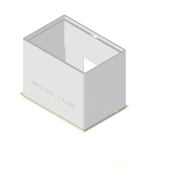
# Autodesk Inventor part: NematostellaImager_v0
Saved by Autodesk Inventor 2022.5 (Build 265521000, 521)
## iProperties
Created: 2023-11-03
Part Number: NematostellaImager_v0
Material: Generisch
Document SubType Name: Modeling
Designer: diederichbenedict
Density: 1 g/cm^3
Appearance: Vorgabe
Author: diederichbenedict
Autodesk Inventor part; units mm, degrees
ref_plane "Arbeitsebene1" through (-165.0574, -46.7107, -74.5227) normal (0, -1, 0) x (1, 0, 0)
sketch "Skizze1" plane through (-165.0574, -46.7107, -74.5227) normal (0, -1, 0) x (1, 0, 0)
  arc A0 (-60.945, 42.8) -> (-63.945, 39.8) centre (-60.945, 39.8) ccw projected
  arc A1 (60.945, -42.8) -> (63.945, -39.8) centre (60.945, -39.8) ccw projected
  line L0 (-61.445, 40.3) -> (61.445, 40.3)
  line L1 (61.445, 40.3) -> (61.445, -40.3)
  line L2 (61.445, -40.3) -> (-61.445, -40.3)
  line L3 (-61.445, -40.3) -> (-61.445, 40.3)
  line L4 (66.445, 45.3) -> (-66.445, 45.3)
  line L5 (-66.445, 45.3) -> (-66.445, -45.3)
  line L6 (-66.445, -45.3) -> (66.445, -45.3)
  line L7 (66.445, -45.3) -> (66.445, 45.3)
  circle A2 centre (14.5, -91.1) radius 3 projected
  circle A3 centre (-20.8, -84.8) radius 3 projected
  circle A4 centre (-14.5, -49.5) radius 3 projected
  circle A5 centre (20.8, -55.8) radius 3 projected
  circle A6 centre (14.5, -49.5) radius 3 projected
  circle A7 centre (-20.8, -55.8) radius 3 projected
  circle A8 centre (-14.5, -91.1) radius 3 projected
  circle A9 centre (20.8, -84.8) radius 3 projected
  line L8 (15, -87.3) -> (-15, -87.3) projected
  arc A10 (15, -87.3) -> (17, -85.3) centre (15, -85.3) ccw projected
  line L9 (17, -85.3) -> (17, -55.3) projected
  arc A11 (17, -55.3) -> (15, -53.3) centre (15, -55.3) ccw projected
  line L10 (-15, -53.3) -> (15, -53.3) projected
  arc A12 (-15, -53.3) -> (-17, -55.3) centre (-15, -55.3) ccw projected
  line L11 (-17, -55.3) -> (-17, -85.3) projected
  arc A13 (-17, -85.3) -> (-15, -87.3) centre (-15, -85.3) ccw projected
  circle A14 centre (21, -91.3) radius 2.5 projected
  circle A15 centre (-21, -49.3) radius 2.5 projected
  circle A16 centre (21, -49.3) radius 2.5 projected
  circle A17 centre (-21, -91.3) radius 2.5 projected
  line L12 (-24.25, -47.3) -> (-24.25, -66.05) projected
  arc A18 (-23, -46.05) -> (-24.25, -47.3) centre (-23, -47.3) ccw projected
  line L13 (-4.25, -46.05) -> (-23, -46.05) projected
  line L14 (-4.25, -43.9226) -> (-4.25, -46.05) projected
  arc A19 (-4.25, -43.9226) -> (-5.0944, -42.9348) centre (-5.25, -43.9226) ccw projected
  arc A20 (-4.9, -40.45) -> (-5.0944, -42.9348) centre (-4.9, -41.7) ccw projected
  line L15 (4.9, -40.45) -> (-4.9, -40.45) projected
  arc A21 (5.0944, -42.9348) -> (4.9, -40.45) centre (4.9, -41.7) ccw projected
  arc A22 (5.0944, -42.9348) -> (4.25, -43.9226) centre (5.25, -43.9226) ccw projected
  line L16 (4.25, -46.05) -> (4.25, -43.9226) projected
  line L17 (23, -46.05) -> (4.25, -46.05) projected
  arc A23 (24.25, -47.3) -> (23, -46.05) centre (23, -47.3) ccw projected
  line L18 (24.25, -64.2875) -> (24.25, -47.3) projected
  arc A24 (24.056, -64.3217) -> (24.25, -64.2875) centre (24.15, -64.2875) ccw projected
  arc A25 (24.056, -64.3217) -> (18.8, -65.25) centre (21.51, -65.25) ccw projected
  line L19 (18.8, -75.35) -> (18.8, -65.25) projected
  arc A26 (18.8, -75.35) -> (24.056, -76.2783) centre (21.51, -75.35) ccw projected
  arc A27 (24.25, -76.3125) -> (24.056, -76.2783) centre (24.15, -76.3125) ccw projected
  line L20 (24.25, -93.3) -> (24.25, -76.3125) projected
  arc A28 (23, -94.55) -> (24.25, -93.3) centre (23, -93.3) ccw projected
  line L21 (6.0125, -94.55) -> (23, -94.55) projected
  arc A29 (5.9783, -94.356) -> (6.0125, -94.55) centre (6.0125, -94.45) ccw projected
  arc A30 (5.9783, -94.356) -> (5.05, -89.1) centre (5.05, -91.81) ccw projected
  line L22 (-5.05, -89.1) -> (5.05, -89.1) projected
  arc A31 (-5.05, -89.1) -> (-5.9783, -94.356) centre (-5.05, -91.81) ccw projected
  arc A32 (-6.0125, -94.55) -> (-5.9783, -94.356) centre (-6.0125, -94.45) ccw projected
  line L23 (-23, -94.55) -> (-6.0125, -94.55) projected
  arc A33 (-24.25, -93.3) -> (-23, -94.55) centre (-23, -93.3) ccw projected
  line L24 (-24.25, -74.55) -> (-24.25, -93.3) projected
  line L25 (-26.3774, -74.55) -> (-24.25, -74.55) projected
  arc A34 (-26.3774, -74.55) -> (-27.3652, -75.3944) centre (-26.3774, -75.55) ccw projected
  arc A35 (-29.85, -75.2) -> (-27.3652, -75.3944) centre (-28.6, -75.2) ccw projected
  line L26 (-29.85, -65.4) -> (-29.85, -75.2) projected
  arc A36 (-27.3652, -65.2056) -> (-29.85, -65.4) centre (-28.6, -65.4) ccw projected
  arc A37 (-27.3652, -65.2056) -> (-26.3774, -66.05) centre (-26.3774, -65.05) ccw projected
  line L27 (-24.25, -66.05) -> (-26.3774, -66.05) projected
  line L28 (-25, -65.3) -> (-25, -47.3) projected
  line L29 (-25, -65.3) -> (-25, -47.3)
  arc A38 (-23, -45.3) -> (-25, -47.3) centre (-23, -47.3) ccw
  line L30 (-23, -45.3) -> (-5, -45.3)
  line L31 (-5, -45.3) -> (-5, -43.9226)
  arc A39 (-5, -43.9226) -> (-5.2111, -43.6757) centre (-5.25, -43.9226) ccw
  arc A40 (-4.9, -39.7) -> (-5.2111, -43.6757) centre (-4.9, -41.7) ccw
  line L32 (-4.9, -39.7) -> (4.9, -39.7)
  arc A41 (5.2111, -43.6757) -> (4.9, -39.7) centre (4.9, -41.7) ccw
  arc A42 (5.2111, -43.6757) -> (5, -43.9226) centre (5.25, -43.9226) ccw
  line L33 (5, -43.9226) -> (5, -45.3)
  line L34 (5, -45.3) -> (23, -45.3)
  arc A43 (25, -47.3) -> (23, -45.3) centre (23, -47.3) ccw
  line L35 (25, -47.3) -> (25, -64.2875)
  arc A44 (23.3514, -64.5786) -> (25, -64.2875) centre (24.15, -64.2875) ccw
  arc A45 (23.3514, -64.5786) -> (19.55, -65.25) centre (21.51, -65.25) ccw
  line L36 (19.55, -65.25) -> (19.55, -75.35)
  arc A46 (19.55, -75.35) -> (23.3514, -76.0214) centre (21.51, -75.35) ccw
  arc A47 (25, -76.3125) -> (23.3514, -76.0214) centre (24.15, -76.3125) ccw
  line L37 (25, -76.3125) -> (25, -93.3)
  arc A48 (23, -95.3) -> (25, -93.3) centre (23, -93.3) ccw
  line L38 (23, -95.3) -> (6.0125, -95.3)
  arc A49 (5.7214, -93.6514) -> (6.0125, -95.3) centre (6.0125, -94.45) ccw
  arc A50 (5.7214, -93.6514) -> (5.05, -89.85) centre (5.05, -91.81) ccw
  line L39 (5.05, -89.85) -> (-5.05, -89.85)
  arc A51 (-5.05, -89.85) -> (-5.7214, -93.6514) centre (-5.05, -91.81) ccw
  arc A52 (-6.0125, -95.3) -> (-5.7214, -93.6514) centre (-6.0125, -94.45) ccw
  line L40 (-6.0125, -95.3) -> (-23, -95.3)
  arc A53 (-25, -93.3) -> (-23, -95.3) centre (-23, -93.3) ccw
  line L41 (-25, -93.3) -> (-25, -75.3)
  line L42 (-25, -75.3) -> (-26.3774, -75.3)
  arc A54 (-26.3774, -75.3) -> (-26.6243, -75.5111) centre (-26.3774, -75.55) ccw
  arc A55 (-30.6, -75.2) -> (-26.6243, -75.5111) centre (-28.6, -75.2) ccw
  line L43 (-30.6, -75.2) -> (-30.6, -65.4)
  arc A56 (-26.6243, -65.0889) -> (-30.6, -65.4) centre (-28.6, -65.4) ccw
  arc A57 (-26.6243, -65.0889) -> (-26.3774, -65.3) centre (-26.3774, -65.05) ccw
  line L44 (-26.3774, -65.3) -> (-25, -65.3)
  point P0 (165.0574, 74.5227)
  point P1 (0, -45.3)
  point P2 (5, -45.3)
  point P3 (-5, -45.3)
  dimension "d0" = 5
  dimension "d16" = 0.5
  dimension "d20" = 0.5
  dimension "d21" = 0.5
  dimension "d22" = 0.5
  constraints: 48 end point, 40 point on circle, 20 centre point, 4 parallel, 2 perpendicular, 1 horizontal, 1 midpoint, 38 other
  measures "d0" distance between parallel lines of L0 L4
  measures "d16" vertical distance of A0.end L0.start
  measures "d20" horizontal distance of L0.start A0.start
  measures "d21" horizontal distance of A1.start L1.end
  measures "d22" vertical distance of A1.end L1.end
extrude "Extrusion1" add sketch "Skizze1" along normal blind 5 contours L3 L2 A40 A39 L31 L6 L5 L4 L7 L33 A42 A41 L1 L0 | L0 L1 L2 A41 L32 A40 L3
sketch "Skizze2" plane through (-165.0574, -46.7107, -74.5227) normal (0, -1, 0) x (1, 0, 0)
  point P0 (165.0574, 74.5227)
sketch "Skizze4" plane through (-165.0574, -46.7107, -74.5227) normal (0, 1, 0) x (1, 0, 0)
  line L0 (-66.445, 45.3) -> (-5, 45.3) projected
  line L1 (-66.445, -45.3) -> (-66.445, 45.3) projected
  line L2 (66.445, -45.3) -> (-66.445, -45.3) projected
  line L3 (66.445, 45.3) -> (66.445, -45.3) projected
  line L4 (-62.445, 43.3) -> (-20, 43.3)
  line L5 (21, 42.3) -> (62.445, 42.3)
  line L6 (62.445, 42.3) -> (62.445, -41.3)
  line L7 (62.445, -41.3) -> (-62.445, -41.3)
  line L8 (-62.445, -41.3) -> (-62.445, 43.3)
  line L9 (-25, 46.3) -> (-25, 43.3)
  line L10 (-4.9, 39.7) -> (4.9, 39.7) projected
  arc A0 (-5.2111, 43.6757) -> (-4.9, 39.7) centre (-4.9, 41.7) ccw projected
  arc A1 (-5.2111, 43.6757) -> (-5, 43.9226) centre (-5.25, 43.9226) ccw projected
  line L11 (-5, 45.3) -> (-5, 43.9226) projected
  line L12 (5, 45.3) -> (66.445, 45.3) projected
  line L13 (5, 43.9226) -> (5, 45.3) projected
  arc A2 (5, 43.9226) -> (5.2111, 43.6757) centre (5.25, 43.9226) ccw projected
  arc A3 (4.9, 39.7) -> (5.2111, 43.6757) centre (4.9, 41.7) ccw projected
  line L14 (-25, 66.3) -> (-25, 48.3)
  line L15 (25, 48.3) -> (25, 65.2875)
  line L16 (25, 48.3) -> (25, 42.3)
  line L17 (-25, 43.3) -> (-25, 46.3)
  point P0 (165.0574, -74.5227)
  point P1 (-25, 45.3)
  point P2 (25, 45.3)
  dimension "d9" = 4
  constraints: 20 end point, 2 perpendicular, 2 point on line, 2 vertical, 1 parallel, 6 other
  measures "d9" distance between parallel lines of L1 L8
ref_plane "Arbeitsebene2" through (-229.0024, 13.2893, -117.3227) normal (0, -1, 0) x (1, 0, 0)
ref_plane "Arbeitsebene3" through (-231.5024, 51.2893, -119.8227) normal (0, 1, 0) x (0, 0, 1)
extrude "Extrusion2" add sketch "Skizze4" along normal up to surface (98 mm away) contours L0 L9 L4 L8 L7 L6 L5 L16 L12 L3 L2 L1
sketch "Skizze5" plane through (-231.5024, 51.2893, -29.2227) normal (0, 1, 0) x (1, 0, 0)
  line L0 (5.5, 2.5) -> (127.39, 2.5) projected
  arc A0 (127.39, 2.5) -> (130.39, 5.5) centre (127.39, 5.5) ccw projected
  line L1 (130.39, 5.5) -> (130.39, 85.1) projected
  arc A1 (130.39, 85.1) -> (127.39, 88.1) centre (127.39, 85.1) ccw projected
  line L2 (127.39, 88.1) -> (5.5, 88.1) projected
  arc A2 (5.5, 88.1) -> (2.5, 85.1) centre (5.5, 85.1) ccw projected
  line L3 (2.5, 85.1) -> (2.5, 5.5) projected
  arc A3 (2.5, 5.5) -> (5.5, 2.5) centre (5.5, 5.5) ccw projected
  line L4 (15.2426, 4) -> (125.89, 4) projected
  arc A4 (13.1213, 4.8787) -> (15.2426, 4) centre (15.2426, 7) ccw projected
  line L5 (13.1213, 4.8787) -> (4.8787, 13.1213) projected
  arc A5 (4, 15.2426) -> (4.8787, 13.1213) centre (7, 15.2426) ccw projected
  line L6 (4, 75.3574) -> (4, 15.2426) projected
  arc A6 (4.8787, 77.4787) -> (4, 75.3574) centre (7, 75.3574) ccw projected
  line L7 (4.8787, 77.4787) -> (13.1213, 85.7213) projected
  arc A7 (15.2426, 86.6) -> (13.1213, 85.7213) centre (15.2426, 83.6) ccw projected
  line L8 (125.89, 86.6) -> (15.2426, 86.6) projected
  arc A8 (128.89, 83.6) -> (125.89, 86.6) centre (125.89, 83.6) ccw projected
  line L9 (128.89, 7) -> (128.89, 83.6) projected
  arc A9 (125.89, 4) -> (128.89, 7) centre (125.89, 7) ccw projected
  line L10 (0, 0) -> (0, 90.6) construction
  line L11 (132.89, 0) -> (0, 0) construction
  line L12 (132.89, 90.6) -> (132.89, 0) construction
  line L13 (91.445, 90.6) -> (132.89, 90.6) construction
  line L14 (91.445, 87.6) -> (91.445, 90.6) construction
  line L15 (128.89, 87.6) -> (91.445, 87.6) construction
  line L16 (128.89, 4) -> (128.89, 87.6) construction
  line L17 (4, 4) -> (128.89, 4) construction
  line L18 (4, 88.6) -> (4, 4) construction
  line L19 (41.445, 88.6) -> (4, 88.6) construction
  line L20 (41.445, 90.6) -> (41.445, 88.6) construction
  line L21 (0, 90.6) -> (41.445, 90.6) construction
  line L22 (0, 90.6) -> (132.89, 90.6)
  line L23 (132.89, 90.6) -> (132.89, 0)
  line L24 (132.89, 0) -> (0, 0)
  line L25 (0, 0) -> (0, 90.6)
  point P0 (231.5024, -29.2227)
  constraints: 8 end point, 2 parallel, 1 horizontal, 1 perpendicular
extrude "Extrusion3" add sketch "Skizze5" along normal blind 5 contours L22 L23 L24 L25
sketch "Skizze6" plane through (-227.5024, 51.2893, -33.2732) normal (0, 1, 0) x (1, 0, 0)
  point P0 (227.5024, -33.2732)
ref_plane "Arbeitsebene4" through (-189.5574, 3.2893, -169.3472) normal (0, 1, 0) x (0, 0, 1)
sketch "Skizze7" plane through (-227.5024, 51.2893, -34.0644) normal (0, 1, 0) x (1, 0, 0)
  arc A0 (-1.5, 0.6583) -> (1.5, -2.3417) centre (1.5, 0.6583) ccw projected
  line L0 (1.5, -2.3417) -> (123.39, -2.3417) projected
  arc A1 (123.39, -2.3417) -> (126.39, 0.6583) centre (123.39, 0.6583) ccw projected
  line L1 (126.39, 0.6583) -> (126.39, 80.2583) projected
  arc A2 (126.39, 80.2583) -> (123.39, 83.2583) centre (123.39, 80.2583) ccw projected
  line L2 (123.39, 83.2583) -> (87.445, 83.2583) projected
  line L3 (87.445, 82.7583) -> (87.445, 83.2583) projected
  line L4 (124.89, 82.7583) -> (87.445, 82.7583) projected
  line L5 (124.89, -0.8417) -> (124.89, 82.7583) projected
  line L6 (0, -0.8417) -> (124.89, -0.8417) projected
  line L7 (-4, -4.8417) -> (128.89, -4.8417) projected
  line L8 (128.89, -4.8417) -> (128.89, 85.7583) projected
  line L9 (128.89, 85.7583) -> (-4, 85.7583) projected
  line L10 (-4, 85.7583) -> (-4, -4.8417) projected
  arc A3 (-1.5, 0.6583) -> (1.5, -2.3417) centre (1.5, 0.6583) ccw projected
  line L11 (-1.5, 0.6583) -> (-1.5, 80.2583) projected
  arc A4 (1.5, 83.2583) -> (-1.5, 80.2583) centre (1.5, 80.2583) ccw projected
  line L12 (1.5, 83.2583) -> (123.39, 83.2583) projected
  arc A5 (126.39, 80.2583) -> (123.39, 83.2583) centre (123.39, 80.2583) ccw projected
  line L13 (126.39, 80.2583) -> (126.39, 0.6583) projected
  arc A6 (123.39, -2.3417) -> (126.39, 0.6583) centre (123.39, 0.6583) ccw projected
  line L14 (123.39, -2.3417) -> (1.5, -2.3417) projected
  line L15 (37.445, 85.7583) -> (37.445, 83.7583) projected
  line L16 (37.445, 83.7583) -> (0, 83.7583) projected
  line L17 (0, 83.7583) -> (0, -0.8417) projected
  line L18 (0, -0.8417) -> (124.89, -0.8417) projected
  line L19 (124.89, -0.8417) -> (124.89, 82.7583) projected
  line L20 (124.89, 82.7583) -> (87.445, 82.7583) projected
  line L21 (87.445, 82.7583) -> (87.445, 85.7583) projected
  line L22 (67.445, 85.7583) -> (87.445, 85.7583) projected
  line L23 (67.445, 84.3809) -> (67.445, 85.7583) projected
  arc A7 (67.445, 84.3809) -> (67.6561, 84.134) centre (67.695, 84.3809) ccw projected
  arc A8 (67.345, 80.1583) -> (67.6561, 84.134) centre (67.345, 82.1583) ccw projected
  line L24 (57.545, 80.1583) -> (67.345, 80.1583) projected
  arc A9 (57.2339, 84.134) -> (57.545, 80.1583) centre (57.545, 82.1583) ccw projected
  arc A10 (57.2339, 84.134) -> (57.445, 84.3809) centre (57.195, 84.3809) ccw projected
  line L25 (57.445, 85.7583) -> (57.445, 84.3809) projected
  line L26 (37.445, 85.7583) -> (57.445, 85.7583) projected
  line L27 (2.445, 3.9583) -> (122.445, 3.9583)
  line L28 (122.445, 3.9583) -> (122.445, 78.9583)
  line L29 (122.445, 78.9583) -> (2.445, 78.9583)
  line L30 (2.445, 78.9583) -> (2.445, 3.9583)
  line L31 (2.445, 3.9583) -> (122.445, 78.9583) construction
  line L32 (122.445, 3.9583) -> (2.445, 78.9583) construction
  arc A11 (0, 82.8564) -> (-1.5, 80.2583) centre (1.5, 80.2583) ccw projected
  line L33 (-1.5, 80.2583) -> (-1.5, 0.6583) projected
  line L34 (0, 82.8564) -> (0, -0.8417) projected
  line L35 (87.445, 83.2583) -> (87.445, 85.7583) projected
  line L36 (37.445, 85.7583) -> (37.445, 83.7583) projected
  line L37 (87.445, 85.7583) -> (37.445, 85.7583)
  line L38 (37.445, 85.7583) -> (37.445, 78.9583)
  line L39 (37.445, 78.9583) -> (87.445, 78.9583)
  line L40 (87.445, 78.9583) -> (87.445, 85.7583)
  line L41 (0, 83.7583) -> (37.445, 83.7583)
  line L42 (37.445, 83.7583) -> (37.445, 78.9583)
  line L43 (37.445, 78.9583) -> (0, 78.9583)
  line L44 (0, 78.9583) -> (0, 83.7583)
  point P0 (227.5024, -34.0644)
  point P1 (62.445, 41.4583)
  point P2 (87.445, 83.2583)
  point P3 (69.0153, 83.2583)
  point P4 (55.8747, 83.2583)
  point P5 (37.445, 84.2583)
  point P6 (37.445, 85.7583)
  point P7 (87.445, 85.7583)
  point P8 (0, 82.8564)
  point P9 (0, -0.8417)
  point P10 (87.445, 83.2583)
  point P11 (67.445, 85.7583)
  point P12 (57.445, 85.7583)
  point P13 (37.445, 83.2583)
  dimension "d23" = 120
  dimension "d24" = 75
  constraints: 28 end point, 6 parallel, 3 horizontal, 3 perpendicular, 2 midpoint, 1 point on line
  measures "d23" distance of L29.end L28.end
  measures "d24" distance of L28.end L27.end
extrude "Extrusion4" add sketch "Skizze7" against normal up to surface (48 mm away) contours A4 L12 L38 L29 L43 L17 | L43 L30 L27 L28 L29 L40 L4 L5 L6 L17 | L38 L15 L9 L25 A10 A9 L12 | L12 A9 L24 A8 L3 L40 L29 L38 | L12 A8 A7 L23 L9 L21
chamfer "Fase1" [suppressed]
sketch "Skizze8" plane through (-231.5024, -51.7107, -119.8227) normal (-1, 0, 0) x (0, 0, 1)
  line L0 (88.1, 61.8529) -> (31.5315, 5.2844) projected
  circle A0 centre (48.2732, 16.3693) radius 1.49
  circle A1 centre (78.2732, 46.3693) radius 1.4
  point P0 (119.8227, 51.7107)
  dimension "d30" = 2.98
  dimension "d31" = 2.8
  dimension "d32" = 4
  dimension "d33" = 4
  dimension "d34" = 30
  constraints: 2 centre point
  measures "d30" diameter of A0
  measures "d31" diameter of A1
  measures "d32" distance from line of A1.centre L0
  measures "d33" distance from line of A0.centre L0
  measures "d34" horizontal distance of A1.centre A0.centre
extrude "Extrusion5" cut sketch "Skizze8" against normal through all
fillet "Rundung1" radius 3 4 edges at (-98.6124, 2.2893, -29.2227) (-231.5024, 2.2893, -29.2227) (-98.6124, 2.2893, -119.8227) (-231.5024, 2.2893, -119.8227)
sketch "Skizze9" plane through (-228.5024, -51.7107, -29.2227) normal (0, 0, 1) x (1, 0, 0)
  line L0 (18.22, 41.0836) -> (111.2722, 41.0836) construction
  line L1 (111.2722, 41.0836) -> (111.2722, 14.2695) construction
  line L2 (111.2722, 14.2695) -> (18.22, 14.2695) construction
  line L3 (18.22, 14.2695) -> (18.22, 41.0836) construction
  line L4 (23.2028, 34.8551) -> (22.2932, 34.8551)
  line L5 (22.2932, 34.8551) -> (19.5942, 40.1147)
  line L6 (19.5942, 40.1147) -> (19.5942, 34.8551)
  line L7 (19.5942, 34.8551) -> (18.8379, 34.8551)
  line L8 (18.8379, 34.8551) -> (18.8379, 40.9551)
  line L9 (18.8379, 40.9551) -> (19.9897, 40.9551)
  line L10 (19.9897, 40.9551) -> (22.4465, 36.1255)
  line L11 (22.4465, 36.1255) -> (22.4465, 40.9551)
  line L12 (22.4465, 40.9551) -> (23.2028, 40.9551)
  line L13 (23.2028, 40.9551) -> (23.2028, 34.8551)
  line L14 (24.4386, 34.8551) -> (24.4386, 40.9551)
  line L15 (24.4386, 40.9551) -> (28.2548, 40.9551)
  line L16 (28.2548, 40.9551) -> (28.2548, 40.2334)
  line L17 (28.2548, 40.2334) -> (25.2493, 40.2334)
  line L18 (25.2493, 40.2334) -> (25.2493, 38.5626)
  line L19 (25.2493, 38.5626) -> (28.0522, 38.5626)
  line L20 (28.0522, 38.5626) -> (28.0522, 37.8408)
  line L21 (28.0522, 37.8408) -> (25.2493, 37.8408)
  line L22 (25.2493, 37.8408) -> (25.2493, 35.5768)
  line L23 (25.2493, 35.5768) -> (28.2548, 35.5768)
  line L24 (28.2548, 35.5768) -> (28.2548, 34.8551)
  line L25 (28.2548, 34.8551) -> (24.4386, 34.8551)
  line L26 (34.3746, 34.8551) -> (33.5639, 34.8551)
  line L27 (33.5639, 34.8551) -> (33.5639, 40.1098)
  line L28 (33.5639, 40.1098) -> (31.9722, 36.5358)
  line L29 (31.9722, 36.5358) -> (31.4779, 36.5358)
  line L30 (31.4779, 36.5358) -> (29.9009, 40.1098)
  line L31 (29.9009, 40.1098) -> (29.9009, 34.8551)
  line L32 (29.9009, 34.8551) -> (29.1446, 34.8551)
  line L33 (29.1446, 34.8551) -> (29.1446, 40.9551)
  line L34 (29.1446, 40.9551) -> (30.2519, 40.9551)
  line L35 (30.2519, 40.9551) -> (31.7744, 37.5591)
  line L36 (31.7744, 37.5591) -> (33.2475, 40.9551)
  line L37 (33.2475, 40.9551) -> (34.3746, 40.9551)
  line L38 (34.3746, 40.9551) -> (34.3746, 34.8551)
  line L39 (34.953, 34.8551) -> (37.0094, 40.9551)
  line L40 (37.0094, 40.9551) -> (38.0079, 40.9551)
  line L41 (38.0079, 40.9551) -> (40.0643, 34.8551)
  line L42 (40.0643, 34.8551) -> (39.2091, 34.8551)
  line L43 (39.2091, 34.8551) -> (38.6555, 36.5605)
  line L44 (38.6555, 36.5605) -> (36.3272, 36.5605)
  line L45 (36.3272, 36.5605) -> (35.7736, 34.8551)
  line L46 (35.7736, 34.8551) -> (34.953, 34.8551)
  line L47 (38.433, 37.2526) -> (37.4889, 40.1246)
  line L48 (37.4889, 40.1246) -> (36.5497, 37.2526)
  line L49 (36.5497, 37.2526) -> (38.433, 37.2526)
  line L50 (42.0663, 34.8551) -> (42.0663, 40.2334)
  line L51 (42.0663, 40.2334) -> (40.0198, 40.2334)
  line L52 (40.0198, 40.2334) -> (40.0198, 40.9551)
  line L53 (40.0198, 40.9551) -> (44.9236, 40.9551)
  line L54 (44.9236, 40.9551) -> (44.9236, 40.2334)
  line L55 (44.9236, 40.2334) -> (42.877, 40.2334)
  line L56 (42.877, 40.2334) -> (42.877, 34.8551)
  line L57 (42.877, 34.8551) -> (42.0663, 34.8551)
  spline S0 degree 2 poles (49.8569, 40.2581) (50.203, 39.8527) (50.5885, 38.6664) (50.5885, 37.9051) knots 0 0 0 1 2 2 2
  spline S1 degree 2 poles (50.5885, 37.9051) (50.5885, 37.1636) (50.2129, 35.9624) (49.8569, 35.557) knots 0 0 0 1 2 2 2
  spline S2 degree 2 poles (49.8569, 35.557) (49.4813, 35.1319) (48.4877, 34.7266) (47.8895, 34.7266) knots 0 0 0 1 2 2 2
  spline S3 degree 2 poles (47.8895, 34.7266) (47.2716, 34.7266) (46.283, 35.1468) (45.9221, 35.557) knots 0 0 0 1 2 2 2
  spline S4 degree 2 poles (45.9221, 35.557) (45.5711, 35.9624) (45.1954, 37.1537) (45.1954, 37.9051) knots 0 0 0 1 2 2 2
  spline S5 degree 2 poles (45.1954, 37.9051) (45.1954, 38.6713) (45.5761, 39.8379) (45.927, 40.2581) knots 0 0 0 1 2 2 2
  spline S6 degree 2 poles (45.927, 40.2581) (46.283, 40.6634) (47.2766, 41.0836) (47.8895, 41.0836) knots 0 0 0 1 2 2 2
  spline S7 degree 2 poles (47.8895, 41.0836) (48.5124, 41.0836) (49.5109, 40.6486) (49.8569, 40.2581) knots 0 0 0 1 2 2 2
  spline S8 degree 2 poles (49.7433, 37.9051) (49.7433, 38.5082) (49.4813, 39.4425) (49.244, 39.7489) knots 0 0 0 1 2 2 2
  spline S9 degree 2 poles (49.244, 39.7489) (49.0018, 40.0653) (48.3196, 40.3817) (47.8945, 40.3817) knots 0 0 0 1 2 2 2
  spline S10 degree 2 poles (47.8945, 40.3817) (47.4545, 40.3817) (46.7921, 40.0752) (46.54, 39.7489) knots 0 0 0 1 2 2 2
  spline S11 degree 2 poles (46.54, 39.7489) (46.2978, 39.4375) (46.0407, 38.4983) (46.0407, 37.9051) knots 0 0 0 1 2 2 2
  spline S12 degree 2 poles (46.0407, 37.9051) (46.0407, 36.7039) (47.0492, 35.4285) (47.8945, 35.4285) knots 0 0 0 1 2 2 2
  spline S13 degree 2 poles (47.8945, 35.4285) (48.7398, 35.4285) (49.7433, 36.7039) (49.7433, 37.9051) knots 0 0 0 1 2 2 2
  spline S14 degree 2 poles (53.1788, 34.7463) (52.5164, 34.7463) (51.5871, 35.0232) (51.1768, 35.2209) knots 0 0 0 1 2 2 2
  line L58 (51.1768, 35.2209) -> (51.1768, 36.2392)
  line L59 (51.1768, 36.2392) -> (51.2361, 36.2392)
  spline S15 degree 2 poles (51.2361, 36.2392) (51.6365, 35.8635) (52.6499, 35.4483) (53.1195, 35.4483) knots 0 0 0 1 2 2 2
  spline S16 degree 2 poles (53.1195, 35.4483) (53.7918, 35.4483) (54.4789, 36.0069) (54.4789, 36.4666) knots 0 0 0 1 2 2 2
  spline S17 degree 2 poles (54.4789, 36.4666) (54.4789, 36.8324) (54.118, 37.2872) (53.7275, 37.4009) knots 0 0 0 1 2 2 2
  spline S18 degree 2 poles (53.7275, 37.4009) (53.4458, 37.48) (52.9762, 37.5887) (52.6252, 37.6777) knots 0 0 0 1 2 2 2
  spline S19 degree 2 poles (52.6252, 37.6777) (52.3088, 37.7617) (51.8095, 38.0138) (51.6168, 38.2165) knots 0 0 0 1 2 2 2
  spline S20 degree 2 poles (51.6168, 38.2165) (51.4289, 38.4192) (51.2213, 38.963) (51.2213, 39.3189) knots 0 0 0 1 2 2 2
  spline S21 degree 2 poles (51.2213, 39.3189) (51.2213, 40.0604) (52.378, 41.0638) (53.2727, 41.0638) knots 0 0 0 1 2 2 2
  spline S22 degree 2 poles (53.2727, 41.0638) (53.7868, 41.0638) (54.6964, 40.8612) (55.0869, 40.6684) knots 0 0 0 1 2 2 2
  line L60 (55.0869, 40.6684) -> (55.0869, 39.6995)
  line L61 (55.0869, 39.6995) -> (55.0276, 39.6995)
  spline S23 degree 2 poles (55.0276, 39.6995) (54.736, 39.9664) (53.8264, 40.3619) (53.3271, 40.3619) knots 0 0 0 1 2 2 2
  spline S24 degree 2 poles (53.3271, 40.3619) (52.7636, 40.3619) (52.0666, 39.833) (52.0666, 39.4029) knots 0 0 0 1 2 2 2
  spline S25 degree 2 poles (52.0666, 39.4029) (52.0666, 39.0173) (52.4769, 38.5576) (52.8625, 38.4538) knots 0 0 0 1 2 2 2
  spline S26 degree 2 poles (52.8625, 38.4538) (53.1195, 38.3846) (53.8659, 38.2066) (54.1131, 38.1325) knots 0 0 0 1 2 2 2
  spline S27 degree 2 poles (54.1131, 38.1325) (54.7409, 37.9397) (55.3242, 37.1636) (55.3242, 36.5951) knots 0 0 0 1 2 2 2
  spline S28 degree 2 poles (55.3242, 36.5951) (55.3242, 36.2343) (55.0326, 35.5422) (54.7706, 35.3) knots 0 0 0 1 2 2 2
  spline S29 degree 2 poles (54.7706, 35.3) (54.4789, 35.0331) (53.7374, 34.7463) (53.1788, 34.7463) knots 0 0 0 1 2 2 2
  line L62 (57.5734, 34.8551) -> (57.5734, 40.2334)
  line L63 (57.5734, 40.2334) -> (55.5269, 40.2334)
  line L64 (55.5269, 40.2334) -> (55.5269, 40.9551)
  line L65 (55.5269, 40.9551) -> (60.4306, 40.9551)
  line L66 (60.4306, 40.9551) -> (60.4306, 40.2334)
  line L67 (60.4306, 40.2334) -> (58.3841, 40.2334)
  line L68 (58.3841, 40.2334) -> (58.3841, 34.8551)
  line L69 (58.3841, 34.8551) -> (57.5734, 34.8551)
  line L70 (61.0485, 34.8551) -> (61.0485, 40.9551)
  line L71 (61.0485, 40.9551) -> (64.8647, 40.9551)
  line L72 (64.8647, 40.9551) -> (64.8647, 40.2334)
  line L73 (64.8647, 40.2334) -> (61.8592, 40.2334)
  line L74 (61.8592, 40.2334) -> (61.8592, 38.5626)
  line L75 (61.8592, 38.5626) -> (64.6621, 38.5626)
  line L76 (64.6621, 38.5626) -> (64.6621, 37.8408)
  line L77 (64.6621, 37.8408) -> (61.8592, 37.8408)
  line L78 (61.8592, 37.8408) -> (61.8592, 35.5768)
  line L79 (61.8592, 35.5768) -> (64.8647, 35.5768)
  line L80 (64.8647, 35.5768) -> (64.8647, 34.8551)
  line L81 (64.8647, 34.8551) -> (61.0485, 34.8551)
  line L82 (69.289, 34.8551) -> (65.7545, 34.8551)
  line L83 (65.7545, 34.8551) -> (65.7545, 40.9551)
  line L84 (65.7545, 40.9551) -> (66.5652, 40.9551)
  line L85 (66.5652, 40.9551) -> (66.5652, 35.5768)
  line L86 (66.5652, 35.5768) -> (69.289, 35.5768)
  line L87 (69.289, 35.5768) -> (69.289, 34.8551)
  line L88 (73.4611, 34.8551) -> (69.9266, 34.8551)
  line L89 (69.9266, 34.8551) -> (69.9266, 40.9551)
  line L90 (69.9266, 40.9551) -> (70.7373, 40.9551)
  line L91 (70.7373, 40.9551) -> (70.7373, 35.5768)
  line L92 (70.7373, 35.5768) -> (73.4611, 35.5768)
  line L93 (73.4611, 35.5768) -> (73.4611, 34.8551)
  line L94 (73.4413, 34.8551) -> (75.4977, 40.9551)
  line L95 (75.4977, 40.9551) -> (76.4962, 40.9551)
  line L96 (76.4962, 40.9551) -> (78.5527, 34.8551)
  line L97 (78.5527, 34.8551) -> (77.6975, 34.8551)
  line L98 (77.6975, 34.8551) -> (77.1438, 36.5605)
  line L99 (77.1438, 36.5605) -> (74.8155, 36.5605)
  line L100 (74.8155, 36.5605) -> (74.2619, 34.8551)
  line L101 (74.2619, 34.8551) -> (73.4413, 34.8551)
  line L102 (76.9214, 37.2526) -> (75.9772, 40.1246)
  line L103 (75.9772, 40.1246) -> (75.038, 37.2526)
  line L104 (75.038, 37.2526) -> (76.9214, 37.2526)
  line L105 (83.8766, 34.8551) -> (81.5137, 34.8551)
  line L106 (81.5137, 34.8551) -> (81.5137, 35.478)
  line L107 (81.5137, 35.478) -> (82.2898, 35.478)
  line L108 (82.2898, 35.478) -> (82.2898, 40.3322)
  line L109 (82.2898, 40.3322) -> (81.5137, 40.3322)
  line L110 (81.5137, 40.3322) -> (81.5137, 40.9551)
  line L111 (81.5137, 40.9551) -> (83.8766, 40.9551)
  line L112 (83.8766, 40.9551) -> (83.8766, 40.3322)
  line L113 (83.8766, 40.3322) -> (83.1005, 40.3322)
  line L114 (83.1005, 40.3322) -> (83.1005, 35.478)
  line L115 (83.1005, 35.478) -> (83.8766, 35.478)
  line L116 (83.8766, 35.478) -> (83.8766, 34.8551)
  line L117 (90.11, 34.8551) -> (89.2993, 34.8551)
  line L118 (89.2993, 34.8551) -> (89.2993, 40.1098)
  line L119 (89.2993, 40.1098) -> (87.7076, 36.5358)
  line L120 (87.7076, 36.5358) -> (87.2133, 36.5358)
  line L121 (87.2133, 36.5358) -> (85.6364, 40.1098)
  line L122 (85.6364, 40.1098) -> (85.6364, 34.8551)
  line L123 (85.6364, 34.8551) -> (84.88, 34.8551)
  line L124 (84.88, 34.8551) -> (84.88, 40.9551)
  line L125 (84.88, 40.9551) -> (85.9873, 40.9551)
  line L126 (85.9873, 40.9551) -> (87.5099, 37.5591)
  line L127 (87.5099, 37.5591) -> (88.983, 40.9551)
  line L128 (88.983, 40.9551) -> (90.11, 40.9551)
  line L129 (90.11, 40.9551) -> (90.11, 34.8551)
  line L130 (90.6884, 34.8551) -> (92.7448, 40.9551)
  line L131 (92.7448, 40.9551) -> (93.7433, 40.9551)
  line L132 (93.7433, 40.9551) -> (95.7997, 34.8551)
  line L133 (95.7997, 34.8551) -> (94.9445, 34.8551)
  line L134 (94.9445, 34.8551) -> (94.3909, 36.5605)
  line L135 (94.3909, 36.5605) -> (92.0626, 36.5605)
  line L136 (92.0626, 36.5605) -> (91.509, 34.8551)
  line L137 (91.509, 34.8551) -> (90.6884, 34.8551)
  line L138 (94.1685, 37.2526) -> (93.2243, 40.1246)
  line L139 (93.2243, 40.1246) -> (92.2851, 37.2526)
  line L140 (92.2851, 37.2526) -> (94.1685, 37.2526)
  spline S30 degree 2 poles (98.9338, 34.7365) (98.2862, 34.7365) (97.2135, 35.1319) (96.8279, 35.5323) knots 0 0 0 1 2 2 2
  spline S31 degree 2 poles (96.8279, 35.5323) (96.4424, 35.9377) (96.0321, 37.1339) (96.0321, 37.91) knots 0 0 0 1 2 2 2
  spline S32 degree 2 poles (96.0321, 37.91) (96.0321, 38.6466) (96.4473, 39.8132) (96.8329, 40.2284) knots 0 0 0 1 2 2 2
  spline S33 degree 2 poles (96.8329, 40.2284) (97.2036, 40.6288) (98.2911, 41.0638) (98.9387, 41.0638) knots 0 0 0 1 2 2 2
  spline S34 degree 2 poles (98.9387, 41.0638) (99.2501, 41.0638) (99.8137, 40.9749) (100.0707, 40.8958) knots 0 0 0 1 2 2 2
  spline S35 degree 2 poles (100.0707, 40.8958) (100.2783, 40.8365) (100.7826, 40.619) (100.9358, 40.5399) knots 0 0 0 1 2 2 2
  line L141 (100.9358, 40.5399) -> (100.9358, 39.5611)
  line L142 (100.9358, 39.5611) -> (100.8666, 39.5611)
  spline S36 degree 2 poles (100.8666, 39.5611) (100.7133, 39.6946) (100.392, 39.9368) (100.0954, 40.0752) knots 0 0 0 1 2 2 2
  spline S37 degree 2 poles (100.0954, 40.0752) (99.8483, 40.1988) (99.2106, 40.3619) (98.8448, 40.3619) knots 0 0 0 1 2 2 2
  spline S38 degree 2 poles (98.8448, 40.3619) (97.9649, 40.3619) (96.8774, 39.0371) (96.8774, 37.9348) knots 0 0 0 1 2 2 2
  spline S39 degree 2 poles (96.8774, 37.9348) (96.8774, 37.3218) (97.1641, 36.4023) (97.436, 36.086) knots 0 0 0 1 2 2 2
  spline S40 degree 2 poles (97.436, 36.086) (97.698, 35.7696) (98.4394, 35.4384) (98.9041, 35.4384) knots 0 0 0 1 2 2 2
  spline S41 degree 2 poles (98.9041, 35.4384) (99.2452, 35.4384) (99.9274, 35.5373) (100.1597, 35.6361) knots 0 0 0 1 2 2 2
  line L143 (100.1597, 35.6361) -> (100.1597, 37.213)
  line L144 (100.1597, 37.213) -> (98.7459, 37.213)
  line L145 (98.7459, 37.213) -> (98.7459, 37.9249)
  line L146 (98.7459, 37.9249) -> (100.9605, 37.9249)
  line L147 (100.9605, 37.9249) -> (100.9605, 35.2604)
  spline S42 degree 2 poles (100.9605, 35.2604) (100.8073, 35.1912) (100.2833, 34.9787) (100.0608, 34.9144) knots 0 0 0 1 2 2 2
  spline S43 degree 2 poles (100.0608, 34.9144) (99.7593, 34.8254) (99.2749, 34.7365) (98.9338, 34.7365) knots 0 0 0 1 2 2 2
  line L148 (101.9788, 34.8551) -> (101.9788, 40.9551)
  line L149 (101.9788, 40.9551) -> (105.795, 40.9551)
  line L150 (105.795, 40.9551) -> (105.795, 40.2334)
  line L151 (105.795, 40.2334) -> (102.7895, 40.2334)
  line L152 (102.7895, 40.2334) -> (102.7895, 38.5626)
  line L153 (102.7895, 38.5626) -> (105.5924, 38.5626)
  line L154 (105.5924, 38.5626) -> (105.5924, 37.8408)
  line L155 (105.5924, 37.8408) -> (102.7895, 37.8408)
  line L156 (102.7895, 37.8408) -> (102.7895, 35.5768)
  line L157 (102.7895, 35.5768) -> (105.795, 35.5768)
  line L158 (105.795, 35.5768) -> (105.795, 34.8551)
  line L159 (105.795, 34.8551) -> (101.9788, 34.8551)
  line L160 (111.4057, 34.8551) -> (110.3527, 34.8551)
  line L161 (110.3527, 34.8551) -> (108.4249, 37.2822)
  line L162 (108.4249, 37.2822) -> (107.4955, 37.2822)
  line L163 (107.4955, 37.2822) -> (107.4955, 34.8551)
  line L164 (107.4955, 34.8551) -> (106.6848, 34.8551)
  line L165 (106.6848, 34.8551) -> (106.6848, 40.9551)
  line L166 (106.6848, 40.9551) -> (108.2568, 40.9551)
  spline S44 degree 2 poles (108.2568, 40.9551) (108.7808, 40.9551) (109.4877, 40.8414) (109.809, 40.6338) knots 0 0 0 1 2 2 2
  spline S45 degree 2 poles (109.809, 40.6338) (110.1303, 40.4262) (110.501, 39.7786) (110.501, 39.2991) knots 0 0 0 1 2 2 2
  spline S46 degree 2 poles (110.501, 39.2991) (110.501, 38.6318) (109.8189, 37.7271) (109.2356, 37.5096) knots 0 0 0 1 2 2 2
  line L167 (109.2356, 37.5096) -> (111.4057, 34.8551)
  spline S47 degree 2 poles (109.6557, 39.2348) (109.6557, 39.5018) (109.4679, 39.9121) (109.2702, 40.0455) knots 0 0 0 1 2 2 2
  spline S48 degree 2 poles (109.2702, 40.0455) (109.0971, 40.1592) (108.6374, 40.2532) (108.3013, 40.2532) knots 0 0 0 1 2 2 2
  line L168 (108.3013, 40.2532) -> (107.4955, 40.2532)
  line L169 (107.4955, 40.2532) -> (107.4955, 37.9595)
  line L170 (107.4955, 37.9595) -> (108.2074, 37.9595)
  spline S49 degree 2 poles (108.2074, 37.9595) (108.5583, 37.9595) (109.1169, 38.0831) (109.3097, 38.2758) knots 0 0 0 1 2 2 2
  spline S50 degree 2 poles (109.3097, 38.2758) (109.4877, 38.4439) (109.6557, 38.9185) (109.6557, 39.2348) knots 0 0 0 1 2 2 2
  point P0 (228.5024, 51.7107)
  constraints: 2 other
extrude "Extrusion6" cut sketch "Skizze9" against normal blind 0.5
sketch "Skizze10" plane through (-165.0574, -46.7107, -74.5227) normal (0, 1, 0) x (1, 0, 0)
  line L0 (-60, -36.5) -> (-60, 38.5) projected
  line L1 (-60, 38.5) -> (60, 38.5) projected
  line L2 (60, 38.5) -> (60, -36.5) projected
  line L3 (60, -36.5) -> (-60, -36.5) projected
  arc A0 (-62.445, 42.3981) -> (-63.945, 39.8) centre (-60.945, 39.8) ccw projected
  line L4 (-63.945, 39.8) -> (-63.945, -39.8) projected
  arc A1 (-63.945, -39.8) -> (-60.945, -42.8) centre (-60.945, -39.8) ccw projected
  line L5 (-60.945, -42.8) -> (60.945, -42.8) projected
  arc A2 (60.945, -42.8) -> (63.945, -39.8) centre (60.945, -39.8) ccw projected
  line L6 (63.945, -39.8) -> (63.945, 39.8) projected
  arc A3 (63.945, 39.8) -> (60.945, 42.8) centre (60.945, 39.8) ccw projected
  line L7 (6.5703, 42.8) -> (60.945, 42.8) projected
  arc A4 (4.9, 39.7) -> (6.5703, 42.8) centre (4.9, 41.7) ccw projected
  line L8 (4.9, 39.7) -> (-4.9, 39.7) projected
  arc A5 (-6.5703, 42.8) -> (-4.9, 39.7) centre (-4.9, 41.7) ccw projected
  line L9 (-60.945, 42.8) -> (-25, 42.8) projected
  arc A6 (-60.945, 42.8) -> (-62.445, 42.3981) centre (-60.945, 39.8) ccw projected
  line L10 (58, 36.5) -> (-58, 36.5)
  line L11 (-58, 36.5) -> (-58, -34.5)
  line L12 (-58, -34.5) -> (58, -34.5)
  line L13 (58, -34.5) -> (58, 36.5)
  line L14 (-25, 42.8) -> (-6.5703, 42.8) projected
  point P0 (165.0574, -74.5227)
  dimension "d40" = 2
  constraints: 8 end point, 3 other
  measures "d40" distance between parallel lines of L1 L10
extrude "Extrusion7" cut sketch "Skizze10" against normal through all contours L13 L12 L11 L10
sketch "Skizze12" plane through (-102.6124, -46.7107, -116.8227) normal (-1, 0, 0) x (0, 0, 1)
  line L0 (84.3929, 57.56) -> (27.8244, 0.9915) projected
  line L1 (39.6164, 11.3693) -> (90.6077, 62.3606) projected
  line L2 (5.3979, -5) -> (69.9374, 59.5396)
  line L3 (69.9374, 59.5396) -> (86.3725, 43.1046)
  line L4 (86.3725, 43.1046) -> (21.8329, -21.435)
  line L5 (21.8329, -21.435) -> (5.3979, -5)
  line L6 (5.3979, -5) -> (86.3725, 43.1046) construction
  line L7 (69.9374, 59.5396) -> (21.8329, -21.435) construction
  line L8 (0, -5) -> (84.6, -5) projected
  line L9 (64.9664, 52.2756) -> (8.3979, -4.2929) projected
  point P0 (116.8227, 46.7107)
  point P1 (45.8852, 19.0523)
  dimension "d49" = 3
  constraints: 12 end point, 3 parallel, 2 midpoint, 2 point on line, 1 perpendicular
  measures "d49" horizontal distance of L9.end L2.start
extrude "Extrusion9" cut sketch "Skizze12" along normal blind 127 and the other way blind 2
sketch "Skizze13" plane through (-231.5024, -51.7107, -116.8227) normal (-1, 0, 0) x (0, 0, 1)
  circle A0 centre (71.9405, 186.7297) radius 1.4 projected
  circle A1 centre (15.77, 186.7297) radius 1.4 projected
  line L0 (98.6077, 122.7297) -> (45.2732, 69.3952) projected
  line L1 (98.6077, 190.7297) -> (98.6077, 122.7297) projected
  line L2 (3.2524, 190.7297) -> (98.6077, 190.7297) projected
  line L3 (3.2524, 182.7297) -> (3.2524, 190.7297) projected
  line L4 (90.6077, 182.7297) -> (3.2524, 182.7297) projected
  line L5 (90.6077, 126.0434) -> (90.6077, 182.7297) projected
  line L6 (39.6164, 75.052) -> (90.6077, 126.0434) projected
  line L7 (45.2732, 69.3952) -> (39.6164, 75.052) projected
  circle A2 centre (75.2732, 105.052) radius 1.4 projected
  circle A3 centre (45.2732, 75.052) radius 1.49 projected
  circle A4 centre (60.2732, 90.052) radius 1.4 projected
  point P0 (116.8227, 51.7107)
hole "Bohrung1" at (-231.5024, 23.3414, -71.5495) at (-231.5024, 38.3414, -56.5495) at (-231.5024, 53.3414, -41.5495) direction (1, 0, 0) diameter 2.8 depth 30 tip angle 118
equation "\"d20\" = d16"
equation "\"d21\" = d16"
equation "\"d22\" = d16"
